Autodesk Fusion 360 part; units mm, degrees
note: some values were not read from the file. Set by a fixed rule: which face or edge a step refers to.
(part 5 of 13)
sketch "Sketch1 (2)" plane through (0, 0, 0) normal (0, 0, 1) x (1, 0, 0) in component "Component"
  spline S0 degree 5 poles (13.78, -0.6782) (13.78, -0.6782) (13.7801, -0.6782) (13.7803, -0.6782) (13.7806, -0.6782) (13.7811, -0.6783) (13.7815, -0.6783) (13.7821, -0.6783) (13.7827, -0.6783) (13.7834, -0.6783) (13.7842, -0.6783) (13.785, -0.6784) (13.7858, -0.6784) (13.7868, -0.6784) (13.7878, -0.6784) (13.7888, -0.6784) (13.7899, -0.6784) (13.7911, -0.6784) (13.7923, -0.6785) (13.7936, -0.6785) (13.795, -0.6785) (13.7964, -0.6785) (13.7978, -0.6785) (13.7993, -0.6785) (13.8009, -0.6785) (13.8025, -0.6784) (13.8042, -0.6784) (13.806, -0.6784) (13.8077, -0.6784) (13.8096, -0.6783) (13.8115, -0.6783) (13.8134, -0.6783) (13.8154, -0.6782) (13.8175, -0.6782) (13.8196, -0.6781) (13.8218, -0.6781) (13.824, -0.678) (13.8262, -0.6779) (13.8286, -0.6778) (13.8309, -0.6778) (13.8333, -0.6777) (13.8358, -0.6776) (13.8383, -0.6775) (13.8409, -0.6773) (13.8435, -0.6772) (13.8462, -0.6771) (13.8489, -0.677) (13.8516, -0.6768) (13.8544, -0.6767) (13.8573, -0.6765) (13.8602, -0.6763) (13.8631, -0.6762) (13.8661, -0.676) (13.8691, -0.6758) (13.8722, -0.6756) (13.8753, -0.6754) (13.8785, -0.6751) (13.8817, -0.6749) (13.885, -0.6747) (13.8883, -0.6744) (13.8917, -0.6742) (13.8951, -0.6739) (13.8985, -0.6736) (13.902, -0.6733) (13.9055, -0.673) (13.9091, -0.6727) (13.9127, -0.6724) (13.9163, -0.6721) (13.92, -0.6717) (13.9238, -0.6714) (13.9275, -0.671) (13.9314, -0.6706) (13.9352, -0.6702) (13.9391, -0.6698) (13.9431, -0.6694) (13.947, -0.669) (13.9511, -0.6686) (13.9551, -0.6681) (13.9592, -0.6676) (13.9634, -0.6672) (13.9675, -0.6667) (13.9718, -0.6662) (13.976, -0.6657) (13.9803, -0.6652) (13.9846, -0.6646) (13.989, -0.6641) (13.9934, -0.6635) (13.9979, -0.663) (14.0024, -0.6624) (14.0069, -0.6618) (14.0114, -0.6612) (14.016, -0.6605) (14.0207, -0.6599) (14.0253, -0.6592) (14.03, -0.6586) (14.0348, -0.6579) (14.0396, -0.6572) (14.0444, -0.6565) (14.0492, -0.6558) (14.0541, -0.655) (14.059, -0.6543) (14.064, -0.6535) (14.069, -0.6527) (14.074, -0.6519) (14.079, -0.6511) (14.0841, -0.6503) (14.0893, -0.6494) (14.0944, -0.6486) (14.0996, -0.6477) (14.1048, -0.6468) (14.1101, -0.6459) (14.1154, -0.645) (14.1207, -0.6441) (14.1261, -0.6431) (14.1315, -0.6422) (14.1369, -0.6412) (14.1423, -0.6402) (14.1478, -0.6392) (14.1533, -0.6382) (14.1589, -0.6371) (14.1645, -0.6361) (14.1701, -0.635) (14.1757, -0.6339) (14.1814, -0.6328) (14.1871, -0.6317) (14.1928, -0.6306) (14.1986, -0.6294) (14.2044, -0.6282) (14.2102, -0.627) (14.2161, -0.6258) (14.222, -0.6246) (14.2279, -0.6234) (14.2338, -0.6221) (14.2398, -0.6209) (14.2458, -0.6196) (14.2518, -0.6183) (14.2579, -0.617) (14.264, -0.6156) (14.2701, -0.6143) (14.2762, -0.6129) (14.2824, -0.6115) (14.2886, -0.6101) (14.2949, -0.6087) (14.3011, -0.6072) (14.3074, -0.6058) (14.3137, -0.6043) (14.3201, -0.6028) (14.3264, -0.6013) (14.3328, -0.5997) (14.3392, -0.5982) (14.3457, -0.5966) (14.3522, -0.595) (14.3587, -0.5934) (14.3652, -0.5918) (14.3718, -0.5902) (14.3783, -0.5885) (14.3849, -0.5868) (14.3916, -0.5852) (14.3982, -0.5834) (14.4049, -0.5817) (14.4116, -0.58) (14.4184, -0.5782) (14.4251, -0.5764) (14.4319, -0.5746) (14.4387, -0.5728) (14.4456, -0.5709) (14.4524, -0.5691) (14.4593, -0.5672) (14.4662, -0.5653) (14.4732, -0.5634) (14.4801, -0.5614) (14.4871, -0.5595) (14.4941, -0.5575) (14.5011, -0.5555) (14.5082, -0.5535) (14.5153, -0.5515) (14.5224, -0.5494) (14.5295, -0.5474) (14.5366, -0.5453) (14.5438, -0.5432) (14.551, -0.541) (14.5582, -0.5389) (14.5655, -0.5367) (14.5727, -0.5345) (14.58, -0.5323) (14.5873, -0.5301) (14.5946, -0.5279) (14.602, -0.5256) (14.6094, -0.5233) (14.6168, -0.521) (14.6242, -0.5187) (14.6316, -0.5163) (14.6391, -0.514) (14.6466, -0.5116) (14.6541, -0.5092) (14.6616, -0.5068) (14.6691, -0.5043) (14.6767, -0.5019) (14.6843, -0.4994) (14.6919, -0.4969) (14.6995, -0.4943) (14.7072, -0.4918) (14.7148, -0.4892) (14.7225, -0.4866) (14.7302, -0.484) (14.738, -0.4814) (14.7457, -0.4788) (14.7535, -0.4761) (14.7613, -0.4734) (14.7691, -0.4707) (14.7769, -0.468) (14.7847, -0.4652) (14.7926, -0.4625) (14.8005, -0.4597) (14.8084, -0.4569) (14.8163, -0.454) (14.8243, -0.4512) (14.8322, -0.4483) (14.8402, -0.4454) (14.8482, -0.4425) (14.8562, -0.4396) (14.8643, -0.4366) (14.8723, -0.4336) (14.8804, -0.4307) (14.8885, -0.4276) (14.8966, -0.4246) (14.9047, -0.4215) (14.9129, -0.4185) (14.921, -0.4154) (14.9292, -0.4122) (14.9374, -0.4091) (14.9456, -0.4059) (14.9539, -0.4027) (14.9621, -0.3995) (14.9704, -0.3963) (14.9787, -0.393) (14.987, -0.3898) (14.9953, -0.3865) (15.0036, -0.3832) (15.012, -0.3798) (15.0203, -0.3765) (15.027, -0.3738) (15.0321, -0.3717) (15.0354, -0.3704) (15.0371, -0.3697) knots 0 0 0 0 0 0 0.00416667 0.00833333 0.0125 0.01666667 0.02083333 0.025 0.02916667 0.03333333 0.0375 0.04166667 0.04583333 0.05 0.05416667 0.05833333 0.0625 0.06666667 0.07083333 0.075 0.07916667 0.08333333 0.0875 0.09166667 0.09583333 0.1 0.10416667 0.10833333 0.1125 0.11666667 0.12083333 0.125 0.12916667 0.13333333 0.1375 0.14166667 0.14583333 0.15 0.15416667 0.15833333 0.1625 0.16666667 0.17083333 0.175 0.17916667 0.18333333 0.1875 0.19166667 0.19583333 0.2 0.20416667 0.20833333 0.2125 0.21666667 0.22083333 0.225 0.22916667 0.23333333 0.2375 0.24166667 0.24583333 0.25 0.25416667 0.25833333 0.2625 0.26666667 0.27083333 0.275 0.27916667 0.28333333 0.2875 0.29166667 0.29583333 0.3 0.30416667 0.30833333 0.3125 0.31666667 0.32083333 0.325 0.32916667 0.33333333 0.3375 0.34166667 0.34583333 0.35 0.35416667 0.35833333 0.3625 0.36666667 0.37083333 0.375 0.37916667 0.38333333 0.3875 0.39166667 0.39583333 0.4 0.40416667 0.40833333 0.4125 0.41666667 0.42083333 0.425 0.42916667 0.43333333 0.4375 0.44166667 0.44583333 0.45 0.45416667 0.45833333 0.4625 0.46666667 0.47083333 0.475 0.47916667 0.48333333 0.4875 0.49166667 0.49583333 0.5 0.50416667 0.50833333 0.5125 0.51666667 0.52083333 0.525 0.52916667 0.53333333 0.5375 0.54166667 0.54583333 0.55 0.55416667 0.55833333 0.5625 0.56666667 0.57083333 0.575 0.57916667 0.58333333 0.5875 0.59166667 0.59583333 0.6 0.60416667 0.60833333 0.6125 0.61666667 0.62083333 0.625 0.62916667 0.63333333 0.6375 0.64166667 0.64583333 0.65 0.65416667 0.65833333 0.6625 0.66666667 0.67083333 0.675 0.67916667 0.68333333 0.6875 0.69166667 0.69583333 0.7 0.70416667 0.70833333 0.7125 0.71666667 0.72083333 0.725 0.72916667 0.73333333 0.7375 0.74166667 0.74583333 0.75 0.75416667 0.75833333 0.7625 0.76666667 0.77083333 0.775 0.77916667 0.78333333 0.7875 0.79166667 0.79583333 0.8 0.80416667 0.80833333 0.8125 0.81666667 0.82083333 0.825 0.82916667 0.83333333 0.8375 0.84166667 0.84583333 0.85 0.85416667 0.85833333 0.8625 0.86666667 0.87083333 0.875 0.87916667 0.88333333 0.8875 0.89166667 0.89583333 0.9 0.90416667 0.90833333 0.9125 0.91666667 0.92083333 0.925 0.92916667 0.93333333 0.9375 0.94166667 0.94583333 0.95 0.95416667 0.95833333 0.9625 0.96666667 0.97083333 0.975 0.97916667 0.98333333 0.9875 0.99166667 0.99583333 1 1 1 1 1 1
  spline S1 degree 5 poles (13.78, 0.6782) (13.78, 0.6782) (13.7801, 0.6782) (13.7803, 0.6782) (13.7806, 0.6782) (13.7811, 0.6783) (13.7815, 0.6783) (13.7821, 0.6783) (13.7827, 0.6783) (13.7834, 0.6783) (13.7842, 0.6783) (13.785, 0.6784) (13.7858, 0.6784) (13.7868, 0.6784) (13.7878, 0.6784) (13.7888, 0.6784) (13.7899, 0.6784) (13.7911, 0.6784) (13.7923, 0.6785) (13.7936, 0.6785) (13.795, 0.6785) (13.7964, 0.6785) (13.7978, 0.6785) (13.7993, 0.6785) (13.8009, 0.6785) (13.8025, 0.6784) (13.8042, 0.6784) (13.806, 0.6784) (13.8077, 0.6784) (13.8096, 0.6783) (13.8115, 0.6783) (13.8134, 0.6783) (13.8154, 0.6782) (13.8175, 0.6782) (13.8196, 0.6781) (13.8218, 0.6781) (13.824, 0.678) (13.8262, 0.6779) (13.8286, 0.6778) (13.8309, 0.6778) (13.8333, 0.6777) (13.8358, 0.6776) (13.8383, 0.6775) (13.8409, 0.6773) (13.8435, 0.6772) (13.8462, 0.6771) (13.8489, 0.677) (13.8516, 0.6768) (13.8544, 0.6767) (13.8573, 0.6765) (13.8602, 0.6763) (13.8631, 0.6762) (13.8661, 0.676) (13.8691, 0.6758) (13.8722, 0.6756) (13.8753, 0.6754) (13.8785, 0.6751) (13.8817, 0.6749) (13.885, 0.6747) (13.8883, 0.6744) (13.8917, 0.6742) (13.8951, 0.6739) (13.8985, 0.6736) (13.902, 0.6733) (13.9055, 0.673) (13.9091, 0.6727) (13.9127, 0.6724) (13.9163, 0.6721) (13.92, 0.6717) (13.9238, 0.6714) (13.9275, 0.671) (13.9314, 0.6706) (13.9352, 0.6702) (13.9391, 0.6698) (13.9431, 0.6694) (13.947, 0.669) (13.9511, 0.6686) (13.9551, 0.6681) (13.9592, 0.6676) (13.9634, 0.6672) (13.9675, 0.6667) (13.9718, 0.6662) (13.976, 0.6657) (13.9803, 0.6652) (13.9846, 0.6646) (13.989, 0.6641) (13.9934, 0.6635) (13.9979, 0.663) (14.0024, 0.6624) (14.0069, 0.6618) (14.0114, 0.6612) (14.016, 0.6605) (14.0207, 0.6599) (14.0253, 0.6592) (14.03, 0.6586) (14.0348, 0.6579) (14.0396, 0.6572) (14.0444, 0.6565) (14.0492, 0.6558) (14.0541, 0.655) (14.059, 0.6543) (14.064, 0.6535) (14.069, 0.6527) (14.074, 0.6519) (14.079, 0.6511) (14.0841, 0.6503) (14.0893, 0.6494) (14.0944, 0.6486) (14.0996, 0.6477) (14.1048, 0.6468) (14.1101, 0.6459) (14.1154, 0.645) (14.1207, 0.6441) (14.1261, 0.6431) (14.1315, 0.6422) (14.1369, 0.6412) (14.1423, 0.6402) (14.1478, 0.6392) (14.1533, 0.6382) (14.1589, 0.6371) (14.1645, 0.6361) (14.1701, 0.635) (14.1757, 0.6339) (14.1814, 0.6328) (14.1871, 0.6317) (14.1928, 0.6306) (14.1986, 0.6294) (14.2044, 0.6282) (14.2102, 0.627) (14.2161, 0.6258) (14.222, 0.6246) (14.2279, 0.6234) (14.2338, 0.6221) (14.2398, 0.6209) (14.2458, 0.6196) (14.2518, 0.6183) (14.2579, 0.617) (14.264, 0.6156) (14.2701, 0.6143) (14.2762, 0.6129) (14.2824, 0.6115) (14.2886, 0.6101) (14.2949, 0.6087) (14.3011, 0.6072) (14.3074, 0.6058) (14.3137, 0.6043) (14.3201, 0.6028) (14.3264, 0.6013) (14.3328, 0.5997) (14.3392, 0.5982) (14.3457, 0.5966) (14.3522, 0.595) (14.3587, 0.5934) (14.3652, 0.5918) (14.3718, 0.5902) (14.3783, 0.5885) (14.3849, 0.5868) (14.3916, 0.5852) (14.3982, 0.5834) (14.4049, 0.5817) (14.4116, 0.58) (14.4184, 0.5782) (14.4251, 0.5764) (14.4319, 0.5746) (14.4387, 0.5728) (14.4456, 0.5709) (14.4524, 0.5691) (14.4593, 0.5672) (14.4662, 0.5653) (14.4732, 0.5634) (14.4801, 0.5614) (14.4871, 0.5595) (14.4941, 0.5575) (14.5011, 0.5555) (14.5082, 0.5535) (14.5153, 0.5515) (14.5224, 0.5494) (14.5295, 0.5474) (14.5366, 0.5453) (14.5438, 0.5432) (14.551, 0.541) (14.5582, 0.5389) (14.5655, 0.5367) (14.5727, 0.5345) (14.58, 0.5323) (14.5873, 0.5301) (14.5946, 0.5279) (14.602, 0.5256) (14.6094, 0.5233) (14.6168, 0.521) (14.6242, 0.5187) (14.6316, 0.5163) (14.6391, 0.514) (14.6466, 0.5116) (14.6541, 0.5092) (14.6616, 0.5068) (14.6691, 0.5043) (14.6767, 0.5019) (14.6843, 0.4994) (14.6919, 0.4969) (14.6995, 0.4943) (14.7072, 0.4918) (14.7148, 0.4892) (14.7225, 0.4866) (14.7302, 0.484) (14.738, 0.4814) (14.7457, 0.4788) (14.7535, 0.4761) (14.7613, 0.4734) (14.7691, 0.4707) (14.7769, 0.468) (14.7847, 0.4652) (14.7926, 0.4625) (14.8005, 0.4597) (14.8084, 0.4569) (14.8163, 0.454) (14.8243, 0.4512) (14.8322, 0.4483) (14.8402, 0.4454) (14.8482, 0.4425) (14.8562, 0.4396) (14.8643, 0.4366) (14.8723, 0.4336) (14.8804, 0.4307) (14.8885, 0.4276) (14.8966, 0.4246) (14.9047, 0.4215) (14.9129, 0.4185) (14.921, 0.4154) (14.9292, 0.4122) (14.9374, 0.4091) (14.9456, 0.4059) (14.9539, 0.4027) (14.9621, 0.3995) (14.9704, 0.3963) (14.9787, 0.393) (14.987, 0.3898) (14.9953, 0.3865) (15.0036, 0.3832) (15.012, 0.3798) (15.0203, 0.3765) (15.027, 0.3738) (15.0321, 0.3717) (15.0354, 0.3704) (15.0371, 0.3697) knots 0 0 0 0 0 0 0.00416667 0.00833333 0.0125 0.01666667 0.02083333 0.025 0.02916667 0.03333333 0.0375 0.04166667 0.04583333 0.05 0.05416667 0.05833333 0.0625 0.06666667 0.07083333 0.075 0.07916667 0.08333333 0.0875 0.09166667 0.09583333 0.1 0.10416667 0.10833333 0.1125 0.11666667 0.12083333 0.125 0.12916667 0.13333333 0.1375 0.14166667 0.14583333 0.15 0.15416667 0.15833333 0.1625 0.16666667 0.17083333 0.175 0.17916667 0.18333333 0.1875 0.19166667 0.19583333 0.2 0.20416667 0.20833333 0.2125 0.21666667 0.22083333 0.225 0.22916667 0.23333333 0.2375 0.24166667 0.24583333 0.25 0.25416667 0.25833333 0.2625 0.26666667 0.27083333 0.275 0.27916667 0.28333333 0.2875 0.29166667 0.29583333 0.3 0.30416667 0.30833333 0.3125 0.31666667 0.32083333 0.325 0.32916667 0.33333333 0.3375 0.34166667 0.34583333 0.35 0.35416667 0.35833333 0.3625 0.36666667 0.37083333 0.375 0.37916667 0.38333333 0.3875 0.39166667 0.39583333 0.4 0.40416667 0.40833333 0.4125 0.41666667 0.42083333 0.425 0.42916667 0.43333333 0.4375 0.44166667 0.44583333 0.45 0.45416667 0.45833333 0.4625 0.46666667 0.47083333 0.475 0.47916667 0.48333333 0.4875 0.49166667 0.49583333 0.5 0.50416667 0.50833333 0.5125 0.51666667 0.52083333 0.525 0.52916667 0.53333333 0.5375 0.54166667 0.54583333 0.55 0.55416667 0.55833333 0.5625 0.56666667 0.57083333 0.575 0.57916667 0.58333333 0.5875 0.59166667 0.59583333 0.6 0.60416667 0.60833333 0.6125 0.61666667 0.62083333 0.625 0.62916667 0.63333333 0.6375 0.64166667 0.64583333 0.65 0.65416667 0.65833333 0.6625 0.66666667 0.67083333 0.675 0.67916667 0.68333333 0.6875 0.69166667 0.69583333 0.7 0.70416667 0.70833333 0.7125 0.71666667 0.72083333 0.725 0.72916667 0.73333333 0.7375 0.74166667 0.74583333 0.75 0.75416667 0.75833333 0.7625 0.76666667 0.77083333 0.775 0.77916667 0.78333333 0.7875 0.79166667 0.79583333 0.8 0.80416667 0.80833333 0.8125 0.81666667 0.82083333 0.825 0.82916667 0.83333333 0.8375 0.84166667 0.84583333 0.85 0.85416667 0.85833333 0.8625 0.86666667 0.87083333 0.875 0.87916667 0.88333333 0.8875 0.89166667 0.89583333 0.9 0.90416667 0.90833333 0.9125 0.91666667 0.92083333 0.925 0.92916667 0.93333333 0.9375 0.94166667 0.94583333 0.95 0.95416667 0.95833333 0.9625 0.96666667 0.97083333 0.975 0.97916667 0.98333333 0.9875 0.99166667 0.99583333 1 1 1 1 1 1
  spline S2 degree 5 poles (13.7794, -0.6782) (13.7794, -0.6782) (13.7795, -0.6782) (13.7796, -0.6782) (13.7796, -0.6782) (13.7797, -0.6782) (13.7798, -0.6782) (13.7799, -0.6782) (13.7799, -0.6782) (13.78, -0.6782) knots 0 0 0 0 0 0 0.2 0.4 0.6 0.8 1 1 1 1 1 1
  spline S3 degree 5 poles (13.7794, 0.6782) (13.7794, 0.6782) (13.7795, 0.6782) (13.7796, 0.6782) (13.7796, 0.6782) (13.7797, 0.6782) (13.7798, 0.6782) (13.7799, 0.6782) (13.7799, 0.6782) (13.78, 0.6782) knots 0 0 0 0 0 0 0.2 0.4 0.6 0.8 1 1 1 1 1 1
  line L0 (0, 0) -> (13.7794, -0.6782)
  line L1 (0, 0) -> (13.7794, 0.6782)
  arc A0 (15.0371, -0.3697) -> (15.0371, 0.3697) centre (0, 0) ccw
  point P0 (13.7816, -0.6783)
  point P1 (13.7843, -0.6783)
  point P2 (13.7881, -0.6784)
  point P3 (13.793, -0.6785)
  point P4 (13.7989, -0.6785)
  point P5 (13.806, -0.6784)
  point P6 (13.8141, -0.6783)
  point P7 (13.8233, -0.678)
  point P8 (13.8336, -0.6777)
  point P9 (13.845, -0.6772)
  point P10 (13.8575, -0.6765)
  point P11 (13.871, -0.6757)
  point P12 (13.8856, -0.6746)
  point P13 (13.9013, -0.6734)
  point P14 (13.918, -0.6719)
  point P15 (13.9358, -0.6702)
  point P16 (13.9547, -0.6682)
  point P17 (13.9746, -0.6659)
  point P18 (13.9956, -0.6632)
  point P19 (14.0176, -0.6603)
  point P20 (14.0407, -0.657)
  point P21 (14.0648, -0.6534)
  point P22 (14.09, -0.6493)
  point P23 (14.1162, -0.6449)
  point P24 (14.1434, -0.64)
  point P25 (14.1716, -0.6347)
  point P26 (14.2009, -0.6289)
  point P27 (14.2312, -0.6227)
  point P28 (14.2624, -0.6159)
  point P29 (14.2947, -0.6087)
  point P30 (14.328, -0.6009)
  point P31 (14.3622, -0.5926)
  point P32 (14.3974, -0.5836)
  point P33 (14.4336, -0.5741)
  point P34 (14.4708, -0.564)
  point P35 (14.5089, -0.5533)
  point P36 (14.5479, -0.542)
  point P37 (14.5879, -0.5299)
  point P38 (14.6288, -0.5172)
  point P39 (14.6706, -0.5038)
  point P40 (14.7133, -0.4897)
  point P41 (14.757, -0.4749)
  point P42 (14.8015, -0.4593)
  point P43 (14.8469, -0.443)
  point P44 (14.8932, -0.4259)
  point P45 (14.9403, -0.408)
  point P46 (14.9883, -0.3892)
  point P47 (13.7816, 0.6783)
  point P48 (13.7843, 0.6783)
  point P49 (13.7881, 0.6784)
  point P50 (13.793, 0.6785)
  point P51 (13.7989, 0.6785)
  point P52 (13.806, 0.6784)
  point P53 (13.8141, 0.6783)
  point P54 (13.8233, 0.678)
  point P55 (13.8336, 0.6777)
  point P56 (13.845, 0.6772)
  point P57 (13.8575, 0.6765)
  point P58 (13.871, 0.6757)
  point P59 (13.8856, 0.6746)
  point P60 (13.9013, 0.6734)
  point P61 (13.918, 0.6719)
  point P62 (13.9358, 0.6702)
  point P63 (13.9547, 0.6682)
  point P64 (13.9746, 0.6659)
  point P65 (13.9956, 0.6632)
  point P66 (14.0176, 0.6603)
  point P67 (14.0407, 0.657)
  point P68 (14.0648, 0.6534)
  point P69 (14.09, 0.6493)
  point P70 (14.1162, 0.6449)
  point P71 (14.1434, 0.64)
  point P72 (14.1716, 0.6347)
  point P73 (14.2009, 0.6289)
  point P74 (14.2312, 0.6227)
  point P75 (14.2624, 0.6159)
  point P76 (14.2947, 0.6087)
  point P77 (14.328, 0.6009)
  point P78 (14.3622, 0.5926)
  point P79 (14.3974, 0.5836)
  point P80 (14.4336, 0.5741)
  point P81 (14.4708, 0.564)
  point P82 (14.5089, 0.5533)
  point P83 (14.5479, 0.542)
  point P84 (14.5879, 0.5299)
  point P85 (14.6288, 0.5172)
  point P86 (14.6706, 0.5038)
  point P87 (14.7133, 0.4897)
  point P88 (14.757, 0.4749)
  point P89 (14.8015, 0.4593)
  point P90 (14.8469, 0.443)
  point P91 (14.8932, 0.4259)
  point P92 (14.9403, 0.408)
  point P93 (14.9883, 0.3892)
sketch "Sketch2" plane through (0, 0, 0) normal (0, 0, 1) x (1, 0, 0) in component "Component"
  circle A0 centre (0, 0) radius 13.2604
extrude "Extrude1" add sketch "Sketch2" along normal blind 5 makes body 1 in component "Component"
extrude "Extrude2" add sketch "Sketch1 (2)" along normal blind 5 separate body makes body 2 in component "Component"
pattern_circular "C-Pattern1" count 36 over 360 about axis through (0, 0, 1.75) along (0, 0, 1) of "Extrude2" makes body 3 at (4.5628, 0.575, 1.6667) makes body 4 at (4.3936, 1.3586, 1.6667) makes body 5 at (3.8649, 2.4924, 1.6667) makes body 6 at (3.3734, 3.1257, 1.6667) makes body 7 at (3.1257, 3.3734, 1.6667) makes body 8 at (2.4924, 3.8649, 1.6667) makes body 9 at (3.5669, 8.478, 3.3333) makes body 10 at (1.0203, 4.4843, 1.6667) makes body 11 at (0.2261, 4.5933, 1.6667) makes body 12 at (-0.575, 4.5628, 1.6667) makes body 13 at (-1.7834, 4.239, 1.6667) makes body 14 at (-2.4924, 3.8649, 1.6667) makes body 15 at (-3.1257, 3.3734, 1.6667) makes body 16 at (-3.3734, 3.1257, 1.6667) makes body 17 at (-3.8649, 2.4924, 1.6667) makes body 18 at (-4.239, 1.7834, 1.6667) makes body 19 at (-4.5628, 0.575, 1.6667) makes body 20 at (-4.5933, 0.2261, 1.6667) makes body 21 at (-4.5628, -0.575, 1.6667) makes body 22 at (-4.3936, -1.3586, 1.6667) makes body 23 at (-4.091, -2.1009, 1.6667) makes body 24 at (-3.3734, -3.1257, 1.6667) makes body 25 at (-3.1257, -3.3734, 1.6667) makes body 26 at (-2.4924, -3.8649, 1.6667) makes body 27 at (-1.3586, -4.3936, 1.6667) makes body 28 at (-0.575, -4.5628, 1.6667) makes body 29 at (-0.2261, -4.5933, 1.6667) makes body 30 at (1.0203, -4.4843, 1.6667) makes body 31 at (1.3586, -4.3936, 1.6667) makes body 32 at (2.4924, -3.8649, 1.6667) makes body 33 at (2.7793, -3.664, 1.6667) makes body 34 at (3.3734, -3.1257, 1.6667) makes body 35 at (3.8649, -2.4924, 1.6667) makes body 36 at (4.239, -1.7834, 1.6667) makes body 37 at (4.4843, -1.0203, 1.6667) in component "Component"
combine "Combine1" operation add target body 1 tool bodies 2 3 4 5 6 7 8 9 10 11 12 13 14 15 16 17 18 19 20 21 22 23 24 25 26 27 28 29 30 31 32 33 34 35 36 37 in component "Component"
sketch "Sketch3" plane through (0, 0, 0) normal (0, 0, 1) x (1, 0, 0) in component "Component"
  line L0 (0, 0) -> (61.4399, 0) construction
  line L1 (61.4399, 0) -> (61.4399, 3) construction
  line L2 (61.4399, 3) -> (0, 3) construction
  line L3 (0, 3) -> (0, 0) construction
  constraint perpendicular L0 L1
  constraint parallel L0 L2
  constraint parallel L1 L3
extrude "Extrude3" cut sketch "Sketch1" against normal blind 6 contours A24 | A25 | A26 | A27 | A28 bodies 1 in component "Component"
extrude "Extrude4" cut sketch "Sketch1" against normal blind 4 contours A29 bodies 1 in component "Component"
component "Component" placed x (1, 0, 0) y (0, 1, 0) z (0, 0, 1) at (0, 0, 0)
component "Component" placed x (1, 0, 0) y (0, 1, 0) z (0, 0, 1) at (0, 34, 0)

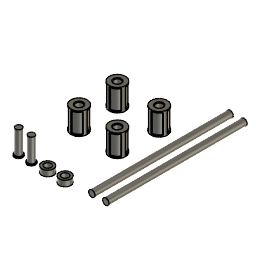
design "card-shuffler-wheels-and-shaft"
part number: 2026-07-30-19-48-15-416
part number: 2026-07-31-16-18-04-707
part number: 2026-07-31-16-25-10-615
part number: 2026-07-31-16-25-10-619
part number: 2026-08-15-23-04-46-105
part number: 2026-08-15-23-04-46-110
part number: 2026-08-17-15-33-29-178
Autodesk Fusion 360 part; units mm, degrees
sketch "Sketch4" plane through (0, 0, 0) normal (0, 0, 1) x (1, 0, 0)
  circle A0 centre (0, 0) radius 6
  circle A1 centre (0, 0) radius 7
  circle A2 centre (35, 0) radius 2.8
  circle A3 centre (0, 0) radius 7.5
  circle A4 centre (35, 0) radius 2.9
  line L0 (0, 0) -> (7, 0)
  line L1 (0, 0) -> (2.8348, 6.4003)
  line L2 (0, 0) -> (-7, 0) construction
  line L3 (0, 0) -> (-6.4003, 2.8348)
  line L4 (0, 0) -> (0, 7)
  line L5 (0, 0) -> (-2.8348, -6.4003)
  line L6 (0, 0) -> (-7, 0)
  line L7 (0, 0) -> (6.4003, -2.8348)
  line L8 (0, 0) -> (0, -7)
  circle A5 centre (0, -45) radius 5
  circle A6 centre (0, -45) radius 2.925
  circle A7 centre (-40, -45) radius 3.5
  dimension "d20" = 12
  dimension "d33" = 5.6
  dimension "d36" = 1
  dimension "d37" = 15
  dimension "d42" = 5.8
  dimension "d44" = 113.889
  dimension "d46" = 360
  dimension "d49" = 5.85
  dimension "d52" = 7
  constraint coincident A0.centre A1.centre
  constraint concentric A2 A4
  constraint coincident A1 L0.end
  constraint horizontal L0
  constraint horizontal L2
  constraint coincident A1 L1.end
  constraint concentric A5 A6
  measures "d20" diameter of A0
  measures "d33" diameter of A2
  measures "d36" distance of A0 A1
  measures "d37" diameter of A3
  measures "d42" diameter of A4
  measures "d44" angle of L1 L2
  measures "d49" diameter of A6
  measures "d52" diameter of A7
extrude "Extrude3" add sketch "Sketch4" along normal blind 19 contours A0 L0 L1 | A0 L0 L7 | A0 L1 L4 | A0 L7 L8 | A0 L3 L6 | A0 L3 L4 | A0 L5 L8 | A0 L5 L6 makes body 1
sketch "Sketch5" plane through (0, 0, 19) normal (0, 0, 1) x (-1, 0, 0)
  circle A0 centre (0, 0) radius 6
  circle A1 centre (0, 0) radius 7
  circle A2 centre (0, 0) radius 2.925
  dimension "d24" = 14
  dimension "d29" = 5.85
  constraint coincident A0.centre A1.centre
  measures "d24" diameter of A1
  measures "d29" diameter of A2
extrude "Extrude5" add sketch "Sketch5" against normal blind 1 contours A1 bodies 1
extrude "Extrude4" add sketch "Sketch4" along normal blind 1 contours A0 A1 L0 L7 | A0 A1 L0 L1 | A0 A1 L1 L4 | A0 A1 L7 L8 | A0 A1 L3 L4 | A0 A1 L5 L8 | A0 A1 L3 L6 | A0 A1 L5 L6 bodies 1
extrude "Extrude6" cut sketch "Sketch5" against normal blind 19 contours A2 bodies 1
chamfer "Chamfer1" distance 0.5 angle 45 2 edges at (2.7271, 1.0577, 0) (2.7271, -1.0577, 19) tangent chain off on bodies 1
extrude "Extrude9" add sketch "Sketch4" along normal blind 19 contours A0 A1 L0 L7 | A0 A1 L1 L4 | A0 A1 L5 L8 | A0 A1 L3 L6 bodies 1
copy_body "Body->Comp2" bodies 1 removing the originals makes body 2 in component "Component"
extrude "Extrude7" add sketch "Sketch4" along normal blind 119 separate body contours A2 makes body 3
copy_body "CopyPasteBodies1" bodies 3 makes body 4
move_body "Move1" bodies 4 to x (1, 0, 0) y (0, 1, 0) z (0, 0, 1) at (-12, 0, 0)
copy_body "Body->Comp3" bodies 3 removing the originals makes body 5 in component "Component'"
copy_body "Body->Comp4" bodies 4 removing the originals makes body 6 in component "Component''"
move_body "Move1'" bodies 6 to x (1, 0, 0) y (0, 0, -1) z (0, 1, 0) at (0, -45, 3) in component "Component''"
move_body "Move1''" bodies 5 to x (1, 0, 0) y (0, 0, -1) z (0, 1, 0) at (0, -45, 3) in component "Component'"
extrude "Extrude10" add sketch "Sketch4" along normal blind 5 separate body contours A5 makes body 7
copy_body "CopyPasteBodies3" bodies 7 makes body 8
move_body "Move4" bodies 8 to x (1, 0, 0) y (0, 1, 0) z (0, 0, 1) at (-15, 0, 0)
copy_body "Body->Comp7" bodies 8 removing the originals makes body 9 in component "Component'''"
copy_body "Body->Comp8" bodies 7 removing the originals makes body 10 in component "Component''''"
extrude "Extrude11" add sketch "Sketch4" along normal blind 1 separate body contours A7 makes body 11
sketch "Sketch6" plane through (0, 0, 1) normal (0, 0, 1) x (-1, 0, 0)
  circle A0 centre (40, 45) radius 3.5
  circle A1 centre (40, 45) radius 2.75
  dimension "d55" = 5.5
  constraint concentric A0 A1
  measures "d55" diameter of A1
extrude "Extrude12" add sketch "Sketch6" along normal blind 20 contours A1 bodies 11
copy_body "Body->Comp9" bodies 11 removing the originals makes body 12 in component "Component'''''"
component "Component" placed x (1, 0, 0) y (0, 1, 0) z (0, 0, 1) at (0, 0, 0)
component "Component" placed x (1, 0, 0) y (0, 1, 0) z (0, 0, 1) at (-33, 0, 0)
component "Component'" placed x (1, 0, 0) y (0, 1, 0) z (0, 0, 1) at (0, 0, 0)
component "Component''" placed x (1, 0, 0) y (0, 1, 0) z (0, 0, 1) at (0, 0, 0)
component "Component" placed x (1, 0, 0) y (0, 1, 0) z (0, 0, 1) at (-34, 34, 0)
component "Component" placed x (1, 0, 0) y (0, 1, 0) z (0, 0, 1) at (2, 34, 0)
component "Component'''" placed x (1, 0, 0) y (0, 1, 0) z (0, 0, 1) at (0, 0, 0)
component "Component''''" placed x (1, 0, 0) y (0, 1, 0) z (0, 0, 1) at (0, 0, 0)
component "Component'''''" placed x (1, 0, 0) y (0, 1, 0) z (0, 0, 1) at (0, 0, 0)
component "Component'''''" placed x (1, 0, 0) y (0, 1, 0) z (0, 0, 1) at (11, 0, 0)
equation "d34 = 93 mm + 20 mm + 6 mm"
equation "d44 = 180 deg - 66.11051484 deg"

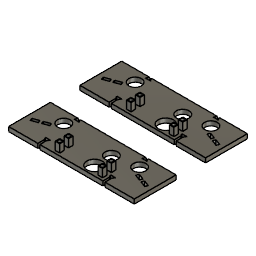
design "card-shuffler-side-plates"
part number: 2026-07-14-13-37-18-342
part number: 2026-07-29-15-30-40-937
Autodesk Fusion 360 part; units mm, degrees
sketch "Sketch1" plane through (0, 0, 0) normal (0, 0, 1) x (1, 0, 0)
  line L0 (0, 0) -> (81, 0)
  line L1 (81, 0) -> (81, 103)
  line L2 (81, 103) -> (0, 103)
  line L3 (0, 103) -> (0, 0)
  line L4 (76, 98) -> (5, 98)
  line L5 (5, 98) -> (5, 5)
  line L6 (5, 5) -> (76, 5)
  line L7 (76, 5) -> (76, 98)
  line L8 (76, 98) -> (5, 5) construction
  line L9 (5, 98) -> (76, 5) construction
  line L10 (81, 0) -> (111, 0)
  line L11 (111, 0) -> (111, 5)
  line L12 (111, 5) -> (81, 5)
  line L13 (81, 5) -> (81, 0)
  line L14 (0, 0) -> (-30, 0)
  line L15 (-30, 0) -> (-30, 5)
  line L16 (-30, 5) -> (0, 5)
  line L17 (0, 5) -> (0, 0)
  line L18 (81, 103) -> (111, 103)
  line L19 (111, 103) -> (111, 98)
  line L20 (111, 98) -> (81, 98)
  line L21 (81, 98) -> (81, 103)
  line L22 (0, 103) -> (-30, 103)
  line L23 (-30, 103) -> (-30, 98)
  line L24 (-30, 98) -> (0, 98)
  line L25 (0, 98) -> (0, 103)
  line L26 (76, 51.5) -> (76, 45)
  line L27 (76, 45) -> (81, 45)
  line L28 (81, 45) -> (81, 58)
  line L29 (81, 58) -> (76, 58)
  line L30 (76, 58) -> (76, 45)
  line L31 (0, 58) -> (5, 58)
  line L32 (5, 58) -> (5, 45)
  line L33 (5, 45) -> (0, 45)
  line L34 (0, 45) -> (0, 58)
  line L35 (81, 98) -> (111, 98)
  line L36 (111, 98) -> (111, 5)
  line L37 (111, 5) -> (81, 5)
  line L38 (81, 5) -> (81, 98)
  line L39 (-30, 98) -> (0, 98)
  line L40 (0, 98) -> (0, 5)
  line L41 (0, 5) -> (-30, 5)
  line L42 (-30, 5) -> (-30, 98)
  line L43 (76, 58) -> (108, 58)
  line L44 (108, 58) -> (108, 45)
  line L45 (108, 45) -> (76, 45)
  line L46 (76, 45) -> (76, 58)
  line L47 (5, 45) -> (-27, 45)
  line L48 (-27, 45) -> (-27, 58)
  line L49 (-27, 58) -> (5, 58)
  line L50 (5, 58) -> (5, 45)
  line L51 (76, 98) -> (81, 98)
  line L52 (5, 98) -> (0, 98)
  line L53 (0, 5) -> (5, 5)
  line L54 (76, 5) -> (81, 5)
  point P0 (40.5, 51.5)
  dimension "d1" = 81
  dimension "d2" = 103
  dimension "d3" = 71
  dimension "d4" = 93
  dimension "d7" = 6.5
  dimension "d8" = 32
  dimension "d9" = 13
  dimension "d14" = 30
  dimension "d15" = 30
  dimension "d16" = 30
  dimension "d17" = 30
  constraint horizontal L0
  constraint vertical L1
  constraint horizontal L2
  constraint vertical L3
  constraint coincident L0.start L3.end
  constraint horizontal L4
  constraint perpendicular L4 L5
  constraint parallel L4 L6
  constraint parallel L5 L7
  constraint coincident L8 P0
  constraint coincident L9 P0
  constraint horizontal L10
  constraint vertical L11
  constraint horizontal L12
  constraint vertical L13
  constraint horizontal L14
  constraint vertical L15
  constraint horizontal L16
  constraint vertical L17
  constraint horizontal L18
  constraint vertical L19
  constraint horizontal L20
  constraint vertical L21
  constraint horizontal L22
  constraint vertical L23
  constraint horizontal L24
  constraint vertical L25
  constraint midpoint L7 L26.start
  constraint parallel L7 L26
  constraint horizontal L27
  constraint vertical L28
  constraint horizontal L29
  constraint vertical L30
  constraint coincident L1 L28.end
  constraint horizontal L31
  constraint vertical L32
  constraint horizontal L33
  constraint vertical L34
  constraint coincident L5 L32.end
  constraint coincident L3 L31.start
  constraint horizontal L35
  constraint vertical L36
  constraint horizontal L37
  constraint vertical L38
  constraint horizontal L39
  constraint vertical L40
  constraint horizontal L41
  constraint vertical L42
  constraint horizontal L43
  constraint vertical L44
  constraint horizontal L45
  constraint vertical L46
  constraint horizontal L47
  constraint vertical L48
  constraint horizontal L49
  constraint vertical L50
  measures "d1" distance of L0.start L0.end
  measures "d2" distance of L0.start L2.end
  measures "d3" distance of L5.end L6.end
  measures "d4" distance of L4.end L5.end
  measures "d7" distance of L26.start L26.end
  measures "d8" distance of L32.end L47.end
  measures "d9" distance of L32.end L31.end
  measures "d14" distance of L36 L38
  measures "d15" distance of L3 L42
  measures "d16" distance of L15 L17
  measures "d17" distance of L19 L21
extrude "Extrude1" add sketch "Sketch1" along normal blind 62 contours L0 L1 L3 L6 L13 L17 L53 L54 | L3 L14 L15 L16 L17 L41 | L1 L10 L11 L12 L13 L37 makes body 1
sketch "Sketch2" plane through (0, 0, 62) normal (0, 0, 1) x (-1, 0, 0)
  line L0 (-76, -98) -> (-81, -98)
  line L1 (-5, -98) -> (0, -98)
  line L2 (0, -5) -> (-5, -5)
  line L3 (40, -98) -> (-121, -98)
  line L4 (-121, -98) -> (-121, -103)
  line L5 (-121, -103) -> (40, -103)
  line L6 (40, -103) -> (40, -98)
  line L7 (40, -5) -> (-121, -5)
  line L8 (-121, -5) -> (-121, 0)
  line L9 (-121, 0) -> (40, 0)
  line L10 (40, 0) -> (40, -5)
  line L11 (0, -5) -> (30, -5)
  line L12 (30, -5) -> (30, 0)
  line L13 (30, 0) -> (-111, 0)
  line L14 (-111, 0) -> (-111, -5)
  line L15 (-111, -5) -> (-81, -5)
  line L16 (-81, -5) -> (-76, -5)
  line L17 (-76, -5) -> (-5, -5)
  line L18 (-5, -5) -> (0, -5)
  constraint horizontal L3
  constraint vertical L4
  constraint horizontal L5
  constraint vertical L6
  constraint horizontal L7
  constraint vertical L8
  constraint horizontal L9
  constraint vertical L10
sketch "Sketch5" plane through (0, 0, 0) normal (0, -1, 0) x (1, 0, 0)
  line L0 (-30, 0) -> (111, 0)
  line L1 (111, 0) -> (111, 62)
  line L2 (111, 62) -> (-30, 62)
  line L3 (-30, 62) -> (-30, 0)
  line L4 (40.5, 62) -> (40.5, 0)
  circle A0 centre (-2, 28) radius 7.05
  circle A1 centre (56, 51.6) radius 8.5
  circle A2 centre (70, 46.6) radius 1.95
  circle A3 centre (70, 56.6) radius 1.95
  line L5 (72.5, 59.1) -> (67.5, 59.1)
  line L6 (67.5, 59.1) -> (67.5, 54.1)
  line L7 (67.5, 54.1) -> (72.5, 54.1)
  line L8 (72.5, 54.1) -> (72.5, 59.1)
  line L9 (72.5, 59.1) -> (67.5, 54.1) construction
  line L10 (67.5, 59.1) -> (72.5, 54.1) construction
  line L11 (72.5, 49.1) -> (67.5, 49.1)
  line L12 (67.5, 49.1) -> (67.5, 44.1)
  line L13 (67.5, 44.1) -> (72.5, 44.1)
  line L14 (72.5, 44.1) -> (72.5, 49.1)
  line L15 (72.5, 49.1) -> (67.5, 44.1) construction
  line L16 (67.5, 49.1) -> (72.5, 44.1) construction
  circle A4 centre (83, 28) radius 7.05
  line L17 (0, 0) -> (80, 0)
  line L18 (80, 0) -> (80, 15)
  line L19 (80, 15) -> (0, 15)
  line L20 (0, 15) -> (0, 0)
  line L21 (0, 15) -> (-30, 15)
  line L22 (-30, 15) -> (-30, 0)
  line L23 (-30, 0) -> (0, 0)
  line L24 (0, 0) -> (0, 15)
  line L25 (80, 15) -> (111, 15)
  line L26 (111, 15) -> (111, 0)
  line L27 (111, 0) -> (80, 0)
  line L28 (80, 0) -> (80, 15)
  line L29 (0, 15) -> (5, 15)
  line L30 (5, 15) -> (5, 18)
  line L31 (5, 18) -> (0, 18)
  line L32 (0, 18) -> (0, 15)
  line L33 (80, 15) -> (75, 15)
  line L34 (81, 18) -> (76, 18)
  line L35 (76, 18) -> (76, 15)
  line L36 (76, 15) -> (81, 15)
  line L37 (81, 15) -> (81, 18)
  line L38 (-7.7431, 38.0574) -> (-14.3209, 40.4516)
  line L39 (-7.7431, 38.0574) -> (-8.7691, 35.2384)
  line L40 (-8.7691, 35.2384) -> (-15.347, 37.6325)
  line L41 (-15.347, 37.6325) -> (-14.3209, 40.4516)
  line L42 (-17.1354, 41.4902) -> (-23.7133, 43.8843)
  line L43 (-17.1354, 41.4902) -> (-18.1615, 38.6711)
  line L44 (-18.1615, 38.6711) -> (-24.7393, 41.0652)
  line L45 (-24.7393, 41.0652) -> (-23.7133, 43.8843)
  line L46 (105.7393, 41.0652) -> (104.7133, 43.8843)
  line L47 (99.1615, 38.6711) -> (105.7393, 41.0652)
  line L48 (96.347, 37.6325) -> (95.3209, 40.4516)
  line L49 (88.7431, 38.0574) -> (95.3209, 40.4516)
  line L50 (98.1354, 41.4902) -> (99.1615, 38.6711)
  line L51 (98.1354, 41.4902) -> (104.7133, 43.8843)
  line L52 (89.7691, 35.2384) -> (96.347, 37.6325)
  line L53 (88.7431, 38.0574) -> (89.7691, 35.2384)
  line L54 (19.5, 59.1) -> (19.5, 54.1)
  line L55 (24.5, 49.1) -> (19.5, 49.1)
  line L56 (24.5, 44.1) -> (24.5, 49.1)
  line L57 (19.5, 44.1) -> (24.5, 44.1)
  line L58 (19.5, 49.1) -> (24.5, 44.1) construction
  line L59 (24.5, 59.1) -> (19.5, 59.1)
  line L60 (24.5, 54.1) -> (24.5, 59.1)
  line L61 (19.5, 54.1) -> (24.5, 54.1)
  line L62 (24.5, 59.1) -> (19.5, 54.1) construction
  circle A5 centre (22, 56.6) radius 1.95
  line L63 (19.5, 49.1) -> (19.5, 44.1)
  line L64 (19.5, 59.1) -> (24.5, 54.1) construction
  circle A6 centre (22, 46.6) radius 1.95
  line L65 (24.5, 49.1) -> (19.5, 44.1) construction
  line L66 (75, 62) -> (75, 36)
  line L67 (104.7133, 43.8843) -> (40.5, 20.5126)
  line L68 (40.5, 20.5126) -> (-23.7133, 43.8843)
  line L69 (62, 62) -> (62, 42)
  circle A7 centre (56, 32.6) radius 7.05
  line L70 (0, 18) -> (2.5, 13.6699)
  line L71 (2.5, 13.6699) -> (5, 18)
  line L72 (5, 18) -> (0, 18)
  line L73 (76, 18) -> (78.5, 13.6699)
  line L74 (78.5, 13.6699) -> (81, 18)
  line L75 (81, 18) -> (76, 18)
  line L76 (5.2598, 18.15) -> (-0.2598, 18.15)
  line L77 (-0.2598, 18.15) -> (2.5, 13.3699)
  line L78 (2.5, 13.3699) -> (5.2598, 18.15)
  line L79 (75.7402, 18.15) -> (78.5, 13.3699)
  line L80 (78.5, 13.3699) -> (81.2598, 18.15)
  line L81 (81.2598, 18.15) -> (75.7402, 18.15)
  point P0 (106, 74)
  point P1 (70, 56.6)
  point P2 (70, 46.6)
  point P3 (22, 46.6)
  point P4 (22, 56.6)
  point P5 (2.5, 16.5566)
  point P6 (78.5, 16.5566)
  dimension "d91" = 14.1
  dimension "d93" = 28
  dimension "d97" = 28
  dimension "d98" = 17
  dimension "d100" = 10.4
  dimension "d101" = 3.9
  dimension "d102" = 3.9
  dimension "d104" = 5
  dimension "d106" = 5
  dimension "d107" = 5
  dimension "d108" = 5
  dimension "d109" = 5
  dimension "d110" = 5
  dimension "d117" = 7
  dimension "d120" = 3
  dimension "d121" = 7
  dimension "d122" = 7
  dimension "d124" = 3
  dimension "d125" = 7
  dimension "d126" = 3
  dimension "d127" = 3.9
  dimension "d128" = 3.9
  dimension "d129" = 5
  dimension "d130" = 5
  dimension "d131" = 5
  dimension "d132" = 5
  dimension "d135" = 3
  dimension "d136" = 3
  dimension "d145" = 14
  dimension "d146" = 14
  dimension "d147" = 14.1
  dimension "d149" = 19
  dimension "d154" = 0.15
  constraint midpoint L2 L4.start
  constraint midpoint L0 L4.end
  constraint horizontal L5
  constraint perpendicular L5 L6
  constraint parallel L5 L7
  constraint parallel L6 L8
  constraint coincident L9 P1
  constraint coincident L10 P1
  constraint coincident P1 A3.centre
  constraint horizontal L11
  constraint perpendicular L11 L12
  constraint parallel L11 L13
  constraint parallel L12 L14
  constraint coincident L15 P2
  constraint coincident L16 P2
  constraint coincident P2 A2.centre
  constraint symmetric L4 A0 A4
  constraint horizontal L17
  constraint vertical L18
  constraint horizontal L19
  constraint vertical L20
  constraint coincident L17.start L20.end
  constraint horizontal L21
  constraint vertical L22
  constraint horizontal L23
  constraint vertical L24
  constraint coincident L0.start L3.end
  constraint horizontal L25
  constraint vertical L26
  constraint horizontal L27
  constraint vertical L28
  constraint coincident L0.end L1.start
  constraint horizontal L29
  constraint vertical L30
  constraint horizontal L31
  constraint vertical L32
  constraint horizontal L33
  constraint horizontal L34
  constraint vertical L35
  constraint horizontal L36
  constraint vertical L37
  constraint coincident L19 L35.end
  constraint perpendicular L38 L39
  constraint perpendicular L39 L40
  constraint perpendicular L41 L42
  constraint perpendicular L42 L43
  constraint perpendicular L43 L44
  constraint symmetric L4 L38.start L49.start
  constraint symmetric L4 L38.end L48.end
  constraint symmetric L4 L39.end L52.start
  constraint symmetric L4 L40.end L48.start
  constraint symmetric L4 L42.start L50.start
  constraint symmetric L4 L42.end L46.end
  constraint symmetric L4 L43.end L47.start
  constraint symmetric L4 L44.end L46.start
  constraint horizontal L59
  constraint perpendicular L54 L59
  constraint parallel L59 L61
  constraint parallel L54 L60
  constraint coincident P4 L62
  constraint coincident P4 L64
  constraint coincident P4 A5.centre
  constraint horizontal L55
  constraint perpendicular L55 L63
  constraint parallel L55 L57
  constraint parallel L56 L63
  constraint coincident P3 L65
  constraint coincident P3 L58
  constraint coincident P3 A6.centre
  constraint coincident L2 L66.start
  constraint perpendicular L2 L66
  constraint coincident L4 L67.end
  constraint perpendicular L48 L67
  constraint coincident L2 L69.start
  constraint perpendicular L2 L69
  measures "d91" diameter of A0
  measures "d93" distance of L0 A0.centre
  measures "d97" distance of L3 A0.centre
  measures "d98" diameter of A1
  measures "d100" distance of L2 A1.centre
  measures "d101" diameter of A2
  measures "d102" diameter of A3
  measures "d104" vertical distance of A1.centre P1
  measures "d106" vertical distance of A1.centre P2
  measures "d107" distance of L6.end L7.end
  measures "d108" distance of L5.end L6.end
  measures "d109" distance of L12.end L13.end
  measures "d110" distance of L11.end L12.end
  measures "d117" distance of L38.start L38.end
  measures "d120" distance of L38.start L39.end
  measures "d121" distance of L39.end L40.end
  measures "d122" distance of L42.start L42.end
  measures "d124" distance of L42.start L43.end
  measures "d125" distance of L43.end L44.end
  measures "d126" distance of L41 L43
  measures "d127" diameter of A6
  measures "d128" diameter of A5
  measures "d129" distance of L54.end L60.start
  measures "d130" distance of L54.end L54.start
  measures "d131" distance of L57.start L56.start
  measures "d132" distance of L55.end L57.start
  measures "d135" distance of L19.end L31.end
  measures "d136" distance of L34.end L35.end
  measures "d145" horizontal distance of A1.centre P1
  measures "d146" horizontal distance of A1.centre P2
  measures "d147" diameter of A7
  measures "d149" distance of A1.centre A7.centre
ref_plane "WorkPlane2" through (40.5, 2.5, 31) normal (1, 0, 0) x (0, 1, 0)
extrude "Extrude13" cut sketch "Sketch5" against normal blind 5 contours L0 L3 L20 L21 L22 L23 L24 | L0 L4 L17 L19 L20 L24 L29 L77 L78 | L0 L4 L17 L18 L19 L28 L33 L36 L79 L80 | L0 L1 L18 L25 L26 L27 L28 L36 | L19 L29 L32 L70 L77 | L19 L29 L70 L71 L77 L78 | L30 L31 L32 L72 L76 L77 L78 | L19 L29 L31 L70 L71 L72 | L19 L29 L70 L71 | L19 L33 L36 L73 L74 L79 L80 | L19 L33 L36 L37 L74 L80 | L19 L29 L30 L71 L78 | L19 L33 L36 L73 L74 | L19 L33 L34 L36 L73 L74 L75 | L34 L35 L37 L75 L79 L80 L81 | L19 L33 L35 L36 L73 L79 | A0 | A1 L69 | A1 L69 | A2 | A3 | L5 L6 L7 L8 | L11 L12 L13 L14 | A4 | L38 L39 L40 L41 | L42 L43 L44 L45 L68 | L46 L47 L50 L51 L67 | L48 L49 L52 L53 | A5 | A6 | L67 A7 | L67 A7 bodies 1
delete_face "DeleteFace1" 4 faces at (76.5196, 5, 15.9) (79.0137, 5, 19.3003) (79.3333, 5, 52.9201) (80.4804, 5, 15.9) on bodies 1
delete_face "DeleteFace2" 1 faces at (1.6667, 5, 52.9201) on bodies 1
copy_body "Body->Comp2" bodies 1 removing the originals makes body 2 in component "Component"
extrude "Extrude2" add sketch "Sketch5" against normal blind 14 contours L5 L6 L7 L8 | L11 L12 L13 L14 | L54 L59 L60 L61 | L55 L56 L57 L63 bodies 2 in component "Component"
sketch "Sketch8" plane through (0, 0, 62) normal (0, 0, 1) x (-1, 0, 0)
  line L0 (-111, -5) -> (30, -5)
  line L1 (30, -5) -> (30, 0)
  line L2 (30, 0) -> (-111, 0)
  line L3 (-81, 0) -> (-76, 0)
  line L4 (-76, 0) -> (-76, -5)
  line L5 (-76, -5) -> (-81, -5)
  line L6 (-81, -5) -> (-81, 0)
  line L7 (0, 0) -> (-5, 0)
  line L8 (-5, 0) -> (-5, -5)
  line L9 (-5, -5) -> (0, -5)
  line L10 (0, -5) -> (0, 0)
  line L11 (-111, 0) -> (-111, -5)
  line L12 (-5, 0) -> (-3, 0)
  line L13 (-3, 0) -> (-3, -5)
  line L14 (-3, -5) -> (-5, -5)
  line L15 (-5, -5) -> (-5, 0)
  line L16 (-76, -5) -> (-78, -5)
  line L17 (-78, -5) -> (-78, 0)
  line L18 (-78, 0) -> (-76, 0)
  line L19 (-76, 0) -> (-76, -5)
  line L20 (-5.5, -5) -> (-2.5, -5)
  line L21 (-2.5, -5) -> (-2.5, 0)
  line L22 (-2.5, 0) -> (-5.5, 0)
  line L23 (-5.5, 0) -> (-5.5, -5)
  line L24 (-5.5, -5) -> (-2.5, 0) construction
  line L25 (-2.5, -5) -> (-5.5, 0) construction
  line L26 (-78.5, -5) -> (-75.5, -5)
  line L27 (-75.5, -5) -> (-75.5, 0)
  line L28 (-75.5, 0) -> (-78.5, 0)
  line L29 (-78.5, 0) -> (-78.5, -5)
  line L30 (-78.5, -5) -> (-75.5, 0) construction
  line L31 (-75.5, -5) -> (-78.5, 0) construction
  line L32 (-75.9, 0) -> (-78.1, 0)
  line L33 (-78.1, 0) -> (-78.1, -5)
  line L34 (-78.1, -5) -> (-75.9, -5)
  line L35 (-75.9, -5) -> (-75.9, 0)
  line L36 (-75.9, 0) -> (-78.1, -5) construction
  line L37 (-78.1, 0) -> (-75.9, -5) construction
  line L38 (-2.9, 0) -> (-5.1, 0)
  line L39 (-5.1, 0) -> (-5.1, -5)
  line L40 (-5.1, -5) -> (-2.9, -5)
  line L41 (-2.9, -5) -> (-2.9, 0)
  line L42 (-2.9, 0) -> (-5.1, -5) construction
  line L43 (-5.1, 0) -> (-2.9, -5) construction
  point P0 (-2.5, -2.5)
  point P1 (-78.5, -2.5)
  point P2 (-4, -2.5)
  point P3 (-77, -2.5)
  point P4 (-77, -2.5)
  point P5 (-4, -2.5)
  constraint horizontal L3
  constraint vertical L4
  constraint horizontal L5
  constraint vertical L6
  constraint coincident L0 L4.end
  constraint coincident L2 L3.start
  constraint horizontal L7
  constraint vertical L8
  constraint horizontal L9
  constraint vertical L10
  constraint coincident L0 L8.end
  constraint coincident L7.start L10.end
  constraint horizontal L12
  constraint vertical L13
  constraint horizontal L14
  constraint vertical L15
  constraint coincident L9 L13.end
  constraint horizontal L16
  constraint vertical L17
  constraint horizontal L18
  constraint vertical L19
  constraint coincident L3 L17.end
  constraint horizontal L20
  constraint perpendicular L20 L21
  constraint parallel L20 L22
  constraint parallel L21 L23
  constraint coincident L24 P5
  constraint coincident L25 P5
  constraint coincident L0 L20.start
  constraint horizontal L26
  constraint perpendicular L26 L27
  constraint parallel L26 L28
  constraint parallel L27 L29
  constraint coincident L30 P4
  constraint coincident L31 P4
  constraint midpoint L5 L26.start
  constraint horizontal L32
  constraint perpendicular L32 L33
  constraint parallel L32 L34
  constraint parallel L33 L35
  constraint coincident L36 P4
  constraint coincident L37 P4
  constraint coincident L28 L32.start
  constraint coincident P4 P3
  constraint horizontal L38
  constraint perpendicular L38 L39
  constraint parallel L38 L40
  constraint parallel L39 L41
  constraint coincident L42 P5
  constraint coincident L43 P5
  constraint coincident L7 L38.start
  constraint coincident P5 P2
extrude "Extrude3" cut sketch "Sketch8" against normal blind 10 contours L0 L2 L3 L5 L17 L26 L28 L32 L33 L34 | L0 L2 L3 L4 L5 L16 L17 L18 L19 L26 L28 L32 L34 | L0 L2 L4 L19 L26 L28 L32 L34 L35 | L0 L2 L8 L15 L20 L22 L38 L39 L40 | L0 L2 L7 L8 L9 L12 L13 L14 L15 L20 L22 L38 L40 | L0 L2 L7 L9 L13 L20 L22 L38 L40 L41 bodies 2 in component "Component"
sketch "Sketch9" plane through (0, 0, 0) normal (0, -1, 0) x (1, 0, 0)
  line L0 (75.9, 62) -> (5.1, 62)
  line L1 (-30, 62) -> (-30, 15)
  line L2 (-30, 15) -> (1.5588, 15)
  line L3 (3.4412, 15) -> (77.5588, 15)
  line L4 (79.4412, 15) -> (111, 15)
  line L5 (111, 15) -> (111, 62)
  line L6 (5.1, 52) -> (2.9, 52)
  line L7 (-15.347, 37.6325) -> (-14.3209, 40.4516)
  line L8 (-14.3209, 40.4516) -> (-7.7431, 38.0574)
  line L9 (-7.7431, 38.0574) -> (-8.7691, 35.2384)
  line L10 (-8.7691, 35.2384) -> (-15.347, 37.6325)
  circle A0 centre (83, 28) radius 7.05
  line L11 (99.1615, 38.6711) -> (98.1354, 41.4902)
  line L12 (98.1354, 41.4902) -> (104.7133, 43.8843)
  line L13 (104.7133, 43.8843) -> (105.7393, 41.0652)
  line L14 (105.7393, 41.0652) -> (99.1615, 38.6711)
  line L15 (-24.7393, 41.0652) -> (-23.7133, 43.8843)
  line L16 (-23.7133, 43.8843) -> (-17.1354, 41.4902)
  line L17 (-17.1354, 41.4902) -> (-18.1615, 38.6711)
  line L18 (-18.1615, 38.6711) -> (-24.7393, 41.0652)
  circle A1 centre (-2, 28) radius 7.05
  line L19 (96.347, 37.6325) -> (89.7691, 35.2384)
  line L20 (89.7691, 35.2384) -> (88.7431, 38.0574)
  line L21 (88.7431, 38.0574) -> (95.3209, 40.4516)
  line L22 (95.3209, 40.4516) -> (96.347, 37.6325)
  circle A2 centre (56, 32.6) radius 7.05
  circle A3 centre (70, 46.6) radius 1.95
  circle A4 centre (22, 46.6) radius 1.95
  line L23 (1.5588, 15) -> (-0.2598, 18.15)
  line L24 (-0.2598, 18.15) -> (5.2598, 18.15)
  line L25 (5.2598, 18.15) -> (3.4412, 15)
  line L26 (77.5588, 15) -> (75.7402, 18.15)
  line L27 (75.7402, 18.15) -> (81.2598, 18.15)
  line L28 (81.2598, 18.15) -> (79.4412, 15)
  circle A5 centre (70, 56.6) radius 1.95
  circle A6 centre (22, 56.6) radius 1.95
  circle A7 centre (56, 51.6) radius 8.5
  line L29 (1.5, 52) -> (6.5, 52)
  line L30 (6.5, 52) -> (4, 56.3301)
  line L31 (4, 56.3301) -> (1.5, 52)
  line L32 (74.5, 52) -> (79.5, 52)
  line L33 (79.5, 52) -> (77, 56.3301)
  line L34 (77, 56.3301) -> (74.5, 52)
  line L35 (79.7598, 51.85) -> (77, 56.6301)
  line L36 (77, 56.6301) -> (74.2402, 51.85)
  line L37 (74.2402, 51.85) -> (79.7598, 51.85)
  line L38 (1.2402, 51.85) -> (6.7598, 51.85)
  line L39 (6.7598, 51.85) -> (4, 56.6301)
  line L40 (4, 56.6301) -> (1.2402, 51.85)
  line L41 (75.9, 52) -> (75.9, 62)
  line L42 (5.1, 62) -> (5.1, 52)
  line L43 (2.9, 52) -> (2.9, 62)
  line L44 (2.9, 62) -> (-30, 62)
  line L45 (111, 62) -> (78.1, 62)
  line L46 (78.1, 62) -> (78.1, 52)
  line L47 (78.1, 52) -> (75.9, 52)
  point P0 (2.5, 53.4434)
  point P1 (78.5, 53.4434)
  point P2 (4, 53.4434)
  point P3 (77, 53.4434)
  dimension "d155" = 0.15
  dimension "d156" = 0.15
extrude "Extrude4" cut sketch "Sketch9" against normal blind 5 contours L32 L33 L34 L35 L36 L37 L41 L46 L47 | L6 L29 L30 L31 L38 L39 L40 L42 L43 | L32 L34 L41 | L29 L30 L42 | L32 L33 L46 | L29 L31 L43 bodies 2 in component "Component"
delete_face "DeleteFace4" 1 faces at (1.9863, 5, 19.3003) on bodies 2 in component "Component"
delete_face "DeleteFace5" 1 faces at (4.4804, 5, 15.9) on bodies 2 in component "Component"
delete_face "DeleteFace6" 1 faces at (0.5196, 5, 15.9) on bodies 2 in component "Component"
component "Component" placed x (1, 0, 0) y (0, 0, 1) z (0, -1, 0) at (0, 34.0061, 0.0547)
component "Component" placed x (1, 0, 0) y (0, 0, 1) z (0, -1, 0) at (0, 114.0061, 0.0547)
equation "d5 = 42.00 mm + 20 mm"

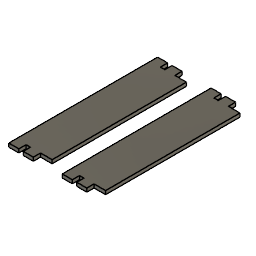
design "card-shuffler-platforms"
part number: 2026-07-28-16-04-37-564
part number: 2026-07-29-15-19-14-329
part number: 2026-07-29-15-19-15-565
Autodesk Fusion 360 part; units mm, degrees